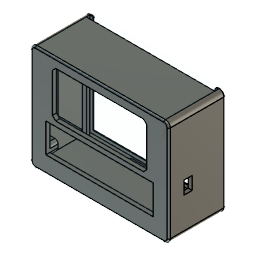
PoDF_A (Autodesk Fusion 360 design; units mm, degrees)
part number: 2026-04-20-19-04-17-052
Autodesk Fusion 360 part; units mm, degrees
note: some values were not read from the file. Set by a fixed rule: which face or edge a step refers to.
sketch "Sketch1" plane through (0, 0, 0) normal (0, 1, 0) x (1, 0, 0)
  line L0 (42.5, 32.5) -> (-42.5, 32.5)
  line L1 (-42.5, 32.5) -> (-42.5, -32.5)
  line L2 (-42.5, -32.5) -> (42.5, -32.5)
  line L3 (42.5, -32.5) -> (42.5, 32.5)
  line L4 (42.5, 32.5) -> (-42.5, -32.5) construction
  line L5 (-42.5, 32.5) -> (42.5, -32.5) construction
  dimension "d1" = 85
  dimension "d2" = 65
  constraint horizontal L0
  constraint perpendicular L0 L1
  constraint parallel L0 L2
  constraint parallel L1 L3
  constraint coincident L4 origin
  constraint coincident L5 origin
  measures "d1" distance of L1.end L2.end
  measures "d2" distance of L0.end L1.end
extrude "Extrude1" add sketch "Sketch1" along normal blind 35
shell "Shell1" thickness 2.5 removed faces 1 at (14.1667, 35, 10.8333)
sketch "Sketch2" plane through (0, 0, 0) normal (0, -1, 0) x (1, 0, 0)
  line L0 (42.5, -32.5) -> (42.5, 32.5)
  line L1 (42.5, 32.5) -> (-42.5, 32.5)
  line L2 (-42.5, 32.5) -> (-42.5, -32.5)
  line L3 (-42.5, -32.5) -> (42.5, -32.5)
sketch "Sketch3" plane through (0, 0, 0) normal (0, -1, 0) x (1, 0, 0)
  line L0 (33, -22) -> (-33, -22)
  line L1 (-33, -22) -> (-33, -4)
  line L2 (-33, -4) -> (33, -4)
  line L3 (33, -4) -> (33, -22)
  line L4 (33, -22) -> (-33, -4) construction
  line L5 (-33, -22) -> (33, -4) construction
  point P0 (0, -13)
  dimension "d7" = 66
  dimension "d8" = 18
  constraint horizontal L0
  constraint perpendicular L0 L1
  constraint parallel L0 L2
  constraint parallel L1 L3
  constraint coincident L4 P0
  constraint coincident L5 P0
  measures "d7" distance of L1.end L2.end
  measures "d8" distance of L0.end L1.end
extrude "Extrude2" cut sketch "Sketch3" against normal up to surface (2.5 mm away)
fillet "Fillet1" radius 3 4 edges at (42.5, 17.5, 32.5) (42.5, 17.5, -32.5) (-42.5, 17.5, 32.5) (-42.5, 17.5, -32.5)
sketch "Sketch4" plane through (0, 0, 0) normal (0, -1, 0) x (1, 0, 0)
  line L0 (29, -1) -> (-29, -1)
  line L1 (-29, -1) -> (-29, 27)
  line L2 (-29, 27) -> (29, 27)
  line L3 (29, 27) -> (29, -1)
  line L4 (29, -1) -> (-29, 27) construction
  line L5 (-29, -1) -> (29, 27) construction
  point P0 (0, 13)
  dimension "d13" = 58
  dimension "d14" = 28
  constraint horizontal L0
  constraint perpendicular L0 L1
  constraint parallel L0 L2
  constraint parallel L1 L3
  constraint coincident L4 P0
  constraint coincident L5 P0
  measures "d13" distance of L1.end L2.end
  measures "d14" distance of L0.end L1.end
extrude "Extrude3" cut sketch "Sketch4" against normal up to surface (2.5 mm away)
sketch "Sketch5" plane through (-40, 0, 0) normal (1, 0, 0) x (0, 1, 0)
  line L0 (2.5, 30) -> (2.5, -30)
  line L1 (2.5, -30) -> (35, -30)
  line L2 (35, -30) -> (35, 30)
  line L3 (35, 30) -> (2.5, 30)
  line L4 (35, -30) -> (29.5, -30)
  line L5 (29.5, -30) -> (29.5, 30)
  line L6 (29.5, 30) -> (35, 30)
  line L7 (35, 30) -> (35, -30)
  dimension "d78" = 27
  constraint horizontal L4
  constraint vertical L5
  constraint horizontal L6
  constraint vertical L7
  constraint coincident L3 L5.end
  constraint coincident L1.end L2.start
  measures "d78" distance of L0 L5
extrude "Extrude4" add sketch "Sketch5" along normal blind 2.5 contours L1 L2 L3 L4 L5 L6 L7
sketch "Sketch6" plane through (40, 0, 0) normal (-1, 0, 0) x (0, -1, 0)
  line L0 (-2.5, -30) -> (-2.5, 30)
  line L1 (-2.5, 30) -> (-35, 30)
  line L2 (-35, 30) -> (-35, -30)
  line L3 (-35, -30) -> (-2.5, -30)
  line L4 (-35, -30) -> (-29.5, -30)
  line L5 (-29.5, -30) -> (-29.5, 30)
  line L6 (-29.5, 30) -> (-35, 30)
  line L7 (-35, 30) -> (-35, -30)
  dimension "d79" = 27
  constraint horizontal L4
  constraint vertical L5
  constraint horizontal L6
  constraint vertical L7
  constraint coincident L1 L5.end
  constraint coincident L2.end L3.start
  measures "d79" distance of L0 L5
extrude "Extrude5" add sketch "Sketch6" along normal blind 2.5 contours L1 L2 L3 L4 L5 L6 L7
sketch "Sketch7" plane through (0, 0, 32.5) normal (0, 0, 1) x (-1, 0, 0)
  line L0 (39.5, -35) -> (39.5, 0)
  line L1 (39.5, 0) -> (-39.5, 0)
  line L2 (-39.5, 0) -> (-39.5, -35)
  line L3 (-39.5, -35) -> (39.5, -35)
sketch "Sketch8" plane through (0, 0, 32.5) normal (0, 0, 1) x (-1, 0, 0)
  line L0 (39.5, -33.5) -> (-39.5, -33.5)
  line L1 (-39.5, -33.5) -> (-39.5, -31.35)
  line L2 (-39.5, -31.35) -> (39.5, -31.35)
  line L3 (39.5, -31.35) -> (39.5, -33.5)
  line L4 (-42.5, 0) -> (42.5, 0)
  dimension "d22" = 2.15
  dimension "d81" = 31.35
  constraint horizontal L0
  constraint vertical L1
  constraint horizontal L2
  constraint vertical L3
  measures "d22" distance of L0.start L2.end
  measures "d81" distance of L2 L4
extrude "Extrude6" cut sketch "Sketch8" against normal up to surface (62.5 mm away)
sketch "Sketch9" plane through (0, 35, 0) normal (0, 1, 0) x (-1, 0, 0)
  line L0 (-37.5, 30) -> (37.5, 30)
  line L1 (37.5, 30) -> (37.5, -30)
  line L2 (37.5, -30) -> (-37.5, -30)
  line L3 (-37.5, -30) -> (-37.5, 30)
  arc A0 (39.5, -32.5) -> (42.5, -29.5) centre (39.5, -29.5) ccw
  line L4 (42.5, -29.5) -> (42.5, 29.5)
  arc A1 (42.5, 29.5) -> (39.5, 32.5) centre (39.5, 29.5) ccw
  line L5 (39.5, 32.5) -> (-39.5, 32.5)
  arc A2 (-39.5, 32.5) -> (-42.5, 29.5) centre (-39.5, 29.5) ccw
  line L6 (-42.5, 29.5) -> (-42.5, -29.5)
  arc A3 (-42.5, -29.5) -> (-39.5, -32.5) centre (-39.5, -29.5) ccw
  line L7 (-39.5, -32.5) -> (39.5, -32.5)
  line L8 (-37.5, 30) -> (37.5, 30)
  line L9 (37.5, 30) -> (37.5, 32.5)
  line L10 (37.5, 32.5) -> (-37.5, 32.5)
  line L11 (-37.5, 32.5) -> (-37.5, 30)
  constraint horizontal L8
  constraint vertical L9
  constraint horizontal L10
  constraint vertical L11
  constraint coincident L5 L9.end
  constraint coincident L0.start L3.end
extrude "Extrude7" cut sketch "Sketch9" against normal up to surface (3.65 mm away) contours L0 L5 L8 L9 L10 L11
sketch "Sketch10" plane through (40, 0, 0) normal (-1, 0, 0) x (0, -1, 0)
  line L0 (-29.5, 30) -> (-29.5, -30)
  line L1 (-29.5, -30) -> (-2.5, -30)
  line L2 (-2.5, -30) -> (-2.5, 30)
  line L3 (-2.5, 30) -> (-29.5, 30)
  line L4 (-2.5, 30) -> (-7.5, 30)
  line L5 (-7.5, 30) -> (-7.5, 24)
  line L6 (-7.5, 24) -> (-2.5, 24)
  line L7 (-2.5, 24) -> (-2.5, 30)
  dimension "d27" = 5
  dimension "d28" = 6
  constraint horizontal L4
  constraint vertical L5
  constraint horizontal L6
  constraint vertical L7
  constraint coincident L2.end L3.start
  measures "d27" distance of L2.end L4.end
  measures "d28" distance of L2.end L6.end
sketch "Sketch12" plane through (0, 2.5, 0) normal (0, 1, 0) x (-1, 0, 0)
  line L0 (-40, 30) -> (-40, -30)
  line L1 (-40, -30) -> (40, -30)
  line L2 (40, -30) -> (40, 30)
  line L3 (40, 30) -> (-40, 30)
  line L4 (-29, -1) -> (-29, 27)
  line L5 (-29, 27) -> (29, 27)
  line L6 (29, 27) -> (29, -1)
  line L7 (29, -1) -> (-29, -1)
  line L8 (-33, -22) -> (-33, -4)
  line L9 (-33, -4) -> (33, -4)
  line L10 (33, -4) -> (33, -22)
  line L11 (33, -22) -> (-33, -22)
  line L12 (-33, -18) -> (-40, -18)
  line L13 (-40, -18) -> (-40, -24)
  line L14 (-40, -24) -> (-33, -24)
  line L15 (-33, -24) -> (-33, -18)
  line L16 (-33, -18) -> (-40, -24) construction
  line L17 (-40, -18) -> (-33, -24) construction
  point P0 (-36.5, -21)
  dimension "d31" = 7
  dimension "d32" = 6
  constraint horizontal L12
  constraint perpendicular L12 L13
  constraint parallel L12 L14
  constraint parallel L13 L15
  constraint coincident L16 P0
  constraint coincident L17 P0
  measures "d31" distance of L13.end L14.end
  measures "d32" distance of L12.end L13.end
extrude "Extrude9" add sketch "Sketch12" along normal blind 5 contours L0 L8 L12 L13 L14 L15
sketch "Sketch13" plane through (0, 2.5, 0) normal (0, 1, 0) x (-1, 0, 0)
  line L0 (-40, -18) -> (-33, -18)
  line L1 (-33, -18) -> (-33, -4)
  line L2 (-33, -4) -> (33, -4)
  line L3 (33, -4) -> (33, -22)
  line L4 (33, -22) -> (-33, -22)
  line L5 (-33, -22) -> (-33, -24)
  line L6 (-33, -24) -> (-40, -24)
  line L7 (-40, -24) -> (-40, -30)
  line L8 (-40, -30) -> (40, -30)
  line L9 (40, -30) -> (40, 30)
  line L10 (40, 30) -> (-40, 30)
  line L11 (-40, 30) -> (-40, -18)
  line L12 (-29, -1) -> (-29, 27)
  line L13 (-29, 27) -> (29, 27)
  line L14 (29, 27) -> (29, -1)
  line L15 (29, -1) -> (-29, -1)
  line L16 (-40, 23) -> (-33, 23)
  line L17 (-33, 23) -> (-33, 17)
  line L18 (-33, 17) -> (-40, 17)
  line L19 (-40, 17) -> (-40, 23)
  dimension "d36" = 35
  constraint horizontal L16
  constraint vertical L17
  constraint horizontal L18
  constraint vertical L19
  constraint coincident L11 L16.start
  measures "d36" distance of L0 L18
extrude "Extrude10" add sketch "Sketch13" along normal blind 5 contours L11 L16 L17 L18 L19
sketch "Sketch14" plane through (0, 2.5, 0) normal (0, 1, 0) x (-1, 0, 0)
  line L0 (-29, -1) -> (-29, 27)
  line L1 (-29, 27) -> (29, 27)
  line L2 (29, 27) -> (29, -1)
  line L3 (29, -1) -> (-29, -1)
  line L4 (-40, 23) -> (-33, 23)
  line L5 (-33, 23) -> (-33, 17)
  line L6 (-33, 17) -> (-40, 17)
  line L7 (-40, 17) -> (-40, -18)
  line L8 (-40, -18) -> (-33, -18)
  line L9 (-33, -18) -> (-33, -4)
  line L10 (-33, -4) -> (33, -4)
  line L11 (33, -4) -> (33, -22)
  line L12 (33, -22) -> (-33, -22)
  line L13 (-33, -22) -> (-33, -24)
  line L14 (-33, -24) -> (-40, -24)
  line L15 (-40, -24) -> (-40, -30)
  line L16 (-40, -30) -> (40, -30)
  line L17 (40, -30) -> (40, 30)
  line L18 (40, 30) -> (-40, 30)
  line L19 (-40, 30) -> (-40, 23)
  line L20 (33, -24) -> (40, -24)
  line L21 (40, -24) -> (40, -18)
  line L22 (40, -18) -> (33, -18)
  line L23 (33, -18) -> (33, -24)
  constraint horizontal L20
  constraint vertical L21
  constraint horizontal L22
  constraint vertical L23
  constraint coincident L17 L21.end
extrude "Extrude11" add sketch "Sketch14" along normal blind 5 contours L11 L17 L20 L21 L22 L23
sketch "Sketch15" plane through (0, 2.5, 0) normal (0, 1, 0) x (-1, 0, 0)
  line L0 (33, -18) -> (40, -18)
  line L1 (40, -18) -> (40, 30)
  line L2 (40, 30) -> (-40, 30)
  line L3 (-40, 30) -> (-40, 23)
  line L4 (-40, 23) -> (-33, 23)
  line L5 (-33, 23) -> (-33, 17)
  line L6 (-33, 17) -> (-40, 17)
  line L7 (-40, 17) -> (-40, -18)
  line L8 (-40, -18) -> (-33, -18)
  line L9 (-33, -18) -> (-33, -4)
  line L10 (-33, -4) -> (33, -4)
  line L11 (33, -4) -> (33, -18)
  line L12 (-29, -1) -> (-29, 27)
  line L13 (-29, 27) -> (29, 27)
  line L14 (29, 27) -> (29, -1)
  line L15 (29, -1) -> (-29, -1)
  line L16 (31, -3) -> (-31, -3)
  line L17 (-31, -3) -> (-31, 29)
  line L18 (-31, 29) -> (31, 29)
  line L19 (31, 29) -> (31, -3)
  line L20 (31, -3) -> (-31, 29) construction
  line L21 (-31, -3) -> (31, 29) construction
  point P0 (0, 13)
  constraint horizontal L16
  constraint perpendicular L16 L17
  constraint parallel L16 L18
  constraint parallel L17 L19
  constraint coincident L20 P0
  constraint coincident L21 P0
extrude "Extrude12" add sketch "Sketch15" along normal blind 2 contours L16 L17 L18 L19
sketch "Sketch16" plane through (0, 4.5, 0) normal (0, 1, 0) x (-1, 0, 0)
  line L0 (29, 27) -> (29, -1)
  line L1 (29, -1) -> (-29, -1)
  line L2 (-29, -1) -> (-29, 27)
  line L3 (-29, 27) -> (29, 27)
  line L4 (31, 29) -> (-31, 29)
  line L5 (-31, 29) -> (-31, -3)
  line L6 (-31, -3) -> (31, -3)
  line L7 (31, -3) -> (31, 29)
  line L8 (30, -2) -> (-30, -2)
  line L9 (-30, -2) -> (-30, 28)
  line L10 (-30, 28) -> (30, 28)
  line L11 (30, 28) -> (30, -2)
  constraint horizontal L8
  constraint vertical L9
  constraint horizontal L10
  constraint vertical L11
extrude "Extrude13" cut sketch "Sketch16" against normal blind 2 contours L8 L9 L10 L11
fillet "Fillet2" radius 2 6 edges at (-33, 5, -18) (-33, 5, -24) (33, 5, -18) (33, 5, -24) (33, 5, 23) (33, 5, 17)
sketch "Sketch17" plane through (40, 0, 0) normal (-1, 0, 0) x (0, -1, 0)
  line L0 (-7.5, 23) -> (-2.5, 23)
  line L1 (-2.5, 23) -> (-2.5, 30)
  line L2 (-2.5, 30) -> (-29.5, 30)
  line L3 (-29.5, 30) -> (-29.5, -30)
  line L4 (-29.5, -30) -> (-2.5, -30)
  line L5 (-2.5, -30) -> (-2.5, -24)
  line L6 (-2.5, -24) -> (-7.5, -24)
  line L7 (-7.5, -24) -> (-7.5, -18)
  line L8 (-7.5, -18) -> (-2.5, -18)
  line L9 (-2.5, -18) -> (-2.5, 17)
  line L10 (-2.5, 17) -> (-7.5, 17)
  line L11 (-7.5, 17) -> (-7.5, 23)
  line L12 (-9.5, -2.5) -> (-14.5, -2.5)
  line L13 (-14.5, -2.5) -> (-14.5, -10.5)
  line L14 (-14.5, -10.5) -> (-9.5, -10.5)
  line L15 (-9.5, -10.5) -> (-9.5, -2.5)
  line L16 (-9.5, -2.5) -> (-14.5, -10.5) construction
  line L17 (-14.5, -2.5) -> (-9.5, -10.5) construction
  point P0 (-12, -6.5)
  dimension "d47" = 5
  dimension "d48" = 8
  dimension "d49" = 23.5
  dimension "d50" = 9.5
  constraint horizontal L12
  constraint perpendicular L12 L13
  constraint parallel L12 L14
  constraint parallel L13 L15
  constraint coincident L16 P0
  constraint coincident L17 P0
  measures "d47" distance of L13.end L14.end
  measures "d48" distance of L12.end L13.end
  measures "d49" distance of L4 P0
  measures "d50" distance of L9 P0
extrude "Extrude14" cut sketch "Sketch17" against normal up to surface (2.5 mm away) contours L12 L13 L14 L15
sketch "Sketch20" plane through (0, 4.5, 0) normal (0, 1, 0) x (-1, 0, 0)
  line L0 (-30, -2) -> (-30, 28)
  line L1 (-30, 28) -> (30, 28)
  line L2 (30, 28) -> (30, -2)
  line L3 (30, -2) -> (-30, -2)
  line L4 (31, 29) -> (-31, 29)
  line L5 (-31, 29) -> (-31, -3)
  line L6 (-31, -3) -> (31, -3)
  line L7 (31, -3) -> (31, 29)
  line L8 (-15, -3) -> (15, -3)
  line L9 (15, -3) -> (15, -2)
  line L10 (15, -2) -> (-15, -2)
  line L11 (-15, -2) -> (-15, -3)
  constraint horizontal L8
  constraint vertical L9
  constraint horizontal L10
  constraint vertical L11
  constraint coincident L3 L9.end
  constraint coincident L6 L8.start
extrude "Extrude15" cut sketch "Sketch20" against normal up to surface (2 mm away) contours L3 L6 L8 L9 L10 L11
sketch "Sketch21" plane through (0, 4.5, 0) normal (0, 1, 0) x (-1, 0, 0)
  line L0 (-15, -3) -> (-15, -2)
  line L1 (-15, -2) -> (-30, -2)
  line L2 (-30, -2) -> (-30, 28)
  line L3 (-30, 28) -> (30, 28)
  line L4 (30, 28) -> (30, -2)
  line L5 (30, -2) -> (15, -2)
  line L6 (15, -2) -> (15, -3)
  line L7 (15, -3) -> (31, -3)
  line L8 (31, -3) -> (31, 29)
  line L9 (31, 29) -> (-31, 29)
  line L10 (-31, 29) -> (-31, -3)
  line L11 (-31, -3) -> (-15, -3)
  line L12 (-15, 28) -> (15, 28)
  line L13 (15, 28) -> (15, 29)
  line L14 (15, 29) -> (-15, 29)
  line L15 (-15, 29) -> (-15, 28)
  constraint horizontal L12
  constraint vertical L13
  constraint horizontal L14
  constraint vertical L15
  constraint coincident L9 L13.end
  constraint coincident L3 L12.start
extrude "Extrude16" cut sketch "Sketch21" against normal up to surface (2 mm away) contours L3 L9 L12 L13 L14 L15
sketch "Sketch22" plane through (0, 2.5, 0) normal (0, 1, 0) x (-1, 0, 0)
  line L0 (15, 29) -> (31, 29)
  line L1 (31, 29) -> (31, -3)
  line L2 (31, -3) -> (15, -3)
  line L3 (15, -3) -> (15, -2)
  line L4 (15, -2) -> (30, -2)
  line L5 (30, -2) -> (30, 28)
  line L6 (30, 28) -> (15, 28)
  line L7 (15, 28) -> (15, 29)
  line L8 (-29, -1) -> (-29, 27)
  line L9 (-29, 27) -> (29, 27)
  line L10 (29, 27) -> (29, -1)
  line L11 (29, -1) -> (-29, -1)
  line L12 (-15, 29) -> (-15, 28)
  line L13 (-15, 28) -> (-30, 28)
  line L14 (-30, 28) -> (-30, -2)
  line L15 (-30, -2) -> (-15, -2)
  line L16 (-15, -2) -> (-15, -3)
  line L17 (-15, -3) -> (-31, -3)
  line L18 (-31, -3) -> (-31, 29)
  line L19 (-31, 29) -> (-15, 29)
  line L20 (35, -18) -> (40, -18)
  line L21 (40, -18) -> (40, 30)
  line L22 (40, 30) -> (-40, 30)
  line L23 (-40, 30) -> (-40, 23)
  line L24 (-40, 23) -> (-35, 23)
  arc A0 (-33, 21) -> (-35, 23) centre (-35, 21) ccw
  line L25 (-33, 21) -> (-33, 19)
  arc A1 (-35, 17) -> (-33, 19) centre (-35, 19) ccw
  line L26 (-35, 17) -> (-40, 17)
  line L27 (-40, 17) -> (-40, -18)
  line L28 (-40, -18) -> (-35, -18)
  arc A2 (-33, -20) -> (-35, -18) centre (-35, -20) ccw
  line L29 (-33, -20) -> (-33, -4)
  line L30 (-33, -4) -> (33, -4)
  line L31 (33, -4) -> (33, -20)
  arc A3 (35, -18) -> (33, -20) centre (35, -20) ccw
  line L32 (27, -1) -> (29, 1)
  line L33 (29, -1) -> (27, -1)
  line L34 (29, 1) -> (29, -1)
  constraint coincident L11 L32.start
  constraint coincident L10 L32.end
  constraint coincident L10.end L11.start
extrude "Extrude17" add sketch "Sketch22" against normal up to surface (2.5 mm away) contours L10 L11 L32 L33 L34
sketch "Sketch23" plane through (0, 2.5, 0) normal (0, 1, 0) x (-1, 0, 0)
  line L0 (15, 29) -> (31, 29)
  line L1 (31, 29) -> (31, -3)
  line L2 (31, -3) -> (15, -3)
  line L3 (15, -3) -> (15, -2)
  line L4 (15, -2) -> (30, -2)
  line L5 (30, -2) -> (30, 28)
  line L6 (30, 28) -> (15, 28)
  line L7 (15, 28) -> (15, 29)
  line L8 (-29, -1) -> (-29, 27)
  line L9 (-29, 27) -> (29, 27)
  line L10 (29, 27) -> (29, 1)
  line L11 (29, 1) -> (27, -1)
  line L12 (27, -1) -> (-29, -1)
  line L13 (-15, 29) -> (-15, 28)
  line L14 (-15, 28) -> (-30, 28)
  line L15 (-30, 28) -> (-30, -2)
  line L16 (-30, -2) -> (-15, -2)
  line L17 (-15, -2) -> (-15, -3)
  line L18 (-15, -3) -> (-31, -3)
  line L19 (-31, -3) -> (-31, 29)
  line L20 (-31, 29) -> (-15, 29)
  line L21 (35, -18) -> (40, -18)
  line L22 (40, -18) -> (40, 30)
  line L23 (40, 30) -> (-40, 30)
  line L24 (-40, 30) -> (-40, 23)
  line L25 (-40, 23) -> (-35, 23)
  arc A0 (-33, 21) -> (-35, 23) centre (-35, 21) ccw
  line L26 (-33, 21) -> (-33, 19)
  arc A1 (-35, 17) -> (-33, 19) centre (-35, 19) ccw
  line L27 (-35, 17) -> (-40, 17)
  line L28 (-40, 17) -> (-40, -18)
  line L29 (-40, -18) -> (-35, -18)
  arc A2 (-33, -20) -> (-35, -18) centre (-35, -20) ccw
  line L30 (-33, -20) -> (-33, -4)
  line L31 (-33, -4) -> (33, -4)
  line L32 (33, -4) -> (33, -20)
  arc A3 (35, -18) -> (33, -20) centre (35, -20) ccw
  line L33 (29, 25) -> (27, 27)
  line L34 (29, 27) -> (27, 27)
  line L35 (29, 27) -> (29, 25)
  line L36 (-29, 27) -> (-27, 27)
  line L37 (-29, 25) -> (-27, 27)
  line L38 (-29, 27) -> (-29, 25)
  line L39 (-29, 1) -> (-27, -1)
  line L40 (-27, -1) -> (-29, -1)
  line L41 (-29, -1) -> (-29, 1)
  constraint coincident L10 L33.start
  constraint coincident L9 L33.end
  constraint coincident L9.end L10.start
  constraint coincident L8.end L9.start
  constraint coincident L9 L36.end
  constraint coincident L8 L37.start
  constraint coincident L8 L39.start
  constraint coincident L12 L39.end
  constraint perpendicular L37 L39
  constraint coincident L8.start L12.end
extrude "Extrude18" add sketch "Sketch23" against normal up to surface (2.5 mm away) contours L8 L12 L39 L40 L41 | L8 L9 L36 L37 L38 | L9 L10 L33 L34 L35
sketch "Sketch26" plane through (0, 7.5, 0) normal (0, 1, 0) x (-1, 0, 0)
  arc A0 (-35, 17) -> (-33, 19) centre (-35, 19) ccw
  line L0 (-33, 19) -> (-33, 21)
  arc A1 (-33, 21) -> (-35, 23) centre (-35, 21) ccw
  line L1 (-35, 23) -> (-40, 23)
  line L2 (-40, 23) -> (-40, 17)
  line L3 (-40, 17) -> (-35, 17)
  circle A2 centre (-36, 20) radius 0.5
  dimension "d65" = 1
  measures "d65" diameter of A2
fillet "Fillet3" radius 1 8 edges at (0, 0, -32.5) (-41.6213, 0, -31.6213) (-42.5, 0, 0) (-41.6213, 0, 31.6213) (0, 0, 32.5) (41.6213, 0, 31.6213) (42.5, 0, 0) (41.6213, 0, -31.6213)
fillet "Fillet4" radius 1 9 edges at (38.5, 35, 32.5) (41.6213, 35, 31.6213) (42.5, 35, 0) (41.6213, 35, -31.6213) (0, 35, -32.5) (-41.6213, 35, -31.6213) (-42.5, 35, 0) (-41.6213, 35, 31.6213) (-38.5, 35, 32.5)
sketch "Sketch27" plane through (0, 0, -30) normal (0, 0, 1) x (-1, 0, 0)
  line L0 (37.5, -31.35) -> (37.5, -29.5)
  line L1 (37.5, -29.5) -> (40, -29.5)
  line L2 (40, -29.5) -> (40, -2.5)
  line L3 (40, -2.5) -> (-40, -2.5)
  line L4 (-40, -2.5) -> (-40, -29.5)
  line L5 (-40, -29.5) -> (-37.5, -29.5)
  line L6 (-37.5, -29.5) -> (-37.5, -31.35)
  line L7 (-37.5, -31.35) -> (-39.5, -31.35)
  line L8 (-39.5, -31.35) -> (-39.5, -33.5)
  line L9 (-39.5, -33.5) -> (-37.5, -33.5)
  line L10 (-37.5, -33.5) -> (-37.5, -35)
  line L11 (-37.5, -35) -> (37.5, -35)
  line L12 (37.5, -35) -> (37.5, -33.5)
  line L13 (37.5, -33.5) -> (39.5, -33.5)
  line L14 (39.5, -33.5) -> (39.5, -31.35)
  line L15 (39.5, -31.35) -> (37.5, -31.35)
  line L16 (37.5, -35) -> (-37.5, -35)
  line L17 (-37.5, -35) -> (-37.5, -33.5)
  line L18 (-37.5, -33.5) -> (37.5, -33.5)
  line L19 (37.5, -33.5) -> (37.5, -35)
  constraint horizontal L16
  constraint vertical L17
  constraint horizontal L18
  constraint vertical L19
  constraint coincident L9.end L10.start
  constraint coincident L11.end L12.start
extrude "Extrude21" add sketch "Sketch27" along normal blind 2 contours L10 L11 L12 L16 L17 L18 L19
fillet "Fillet6" radius 1 7 edges at (-37.5, 35, 1.75) (-37.5, 34.7071, 32.2071) (-37.5, 33.75, 32.5) (0, 35, -28) (37.5, 35, 1.75) (37.5, 34.7071, 32.2071) (37.5, 33.75, 32.5)
hole "Hole1" at (-36, 7.5, -21) direction (0, -1, 0) diameter 0.769 depth 4 tip angle 118
thread "Thread1" "ISO Metric profile 1.0 M1x0.25 M1x0.25 6H" thread offset 0 thread depth 7.4
hole "Hole2" at (36, 7.5, -21) direction (0, -1, 0) diameter 0.769 depth 4 tip angle 118
thread "Thread2" "ISO Metric profile 1.0 M1x0.25 M1x0.25 6H" thread offset 0 thread depth 7.4
hole "Hole3" at (36, 7.5, 20) direction (0, -1, 0) diameter 0.769 depth 4 tip angle 118
thread "Thread3" "ISO Metric profile 1.0 M1x0.25 M1x0.25 6H" thread offset 0 thread depth 7.4
